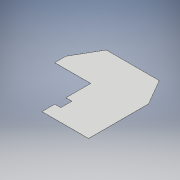
# Autodesk Inventor part: cover 3
Saved by Autodesk Inventor 2018 (Build 220112000, 112)
## iProperties
Created: 2018-03-20
Part Number: cover 3
Material: Generic
Document SubType Name: Modeling
Designer: P446509
Density: 1 g/cm^3
Appearance: Default
Author: P446509
Autodesk Inventor part; units mm, degrees
ref_plane "YZ Plane" through (0, 0, 0) normal (1, 0, 0) x (0, 1, 0)
ref_plane "XZ Plane" through (0, 0, 0) normal (0, 1, 0) x (-1, 0, 0)
ref_plane "XY Plane" through (0, 0, 0) normal (0, 0, 1) x (1, 0, 0)
sketch "Sketch1" plane through (0, 0, 0) normal (0, 0, 1) x (1, 0, 0)
  line L0 (0, 0) -> (385, 0)
  line L1 (385, 0) -> (385, 700)
  line L2 (385, 700) -> (212, 999.6448)
  line L3 (385, 700) -> (731, 700) construction
  line L4 (212, 999.6448) -> (-408, 999.6448)
  line L5 (-408, 999.6448) -> (-581, 700)
  line L6 (0, 0) -> (-160, 0)
  line L7 (-160, 0) -> (-160, 150)
  line L8 (-160, 150) -> (-90, 150)
  line L9 (-90, 150) -> (-90, 280)
  line L10 (-90, 280) -> (-160, 280)
  line L11 (-160, 280) -> (-160, 570)
  line L12 (-581, 700) -> (-581, 570)
  line L13 (-160, 570) -> (-581, 570)
  dimension "d0" = 385
  dimension "d1" = 700
  dimension "d2" = 346
  dimension "d3" = 120
  dimension "d4" = 620
  dimension "d5" = 346
  dimension "d6" = 120
  dimension "d7" = 160
  dimension "d8" = 150
  dimension "d9" = 70
  dimension "d10" = 130
  dimension "d11" = 70
  dimension "d12" = 290
  constraints: 28 end point, 4 horizontal, 4 perpendicular, 3 vertical, 1 equal length, 1 point on line
  measures "d0" distance of L0.start L0.end
  measures "d1" distance of L0.end L1.end
  measures "d2" distance of L1.end L2.end
  measures "d3" angle of L3 L2
  measures "d4" distance of L2.end L4.end
  measures "d5" distance of L4.end L5.end
  measures "d6" angle of L5 L4
  measures "d7" distance of L0.start L6.end
  measures "d8" distance of L6.end L7.end
  measures "d9" distance of L7.end L8.end
  measures "d10" distance of L8.end L9.end
  measures "d11" distance of L9.end L10.end
  measures "d12" distance of L10.end L11.end
extrude "Extrusion1" add sketch "Sketch1" along normal blind 1.6
body "Solid1"
